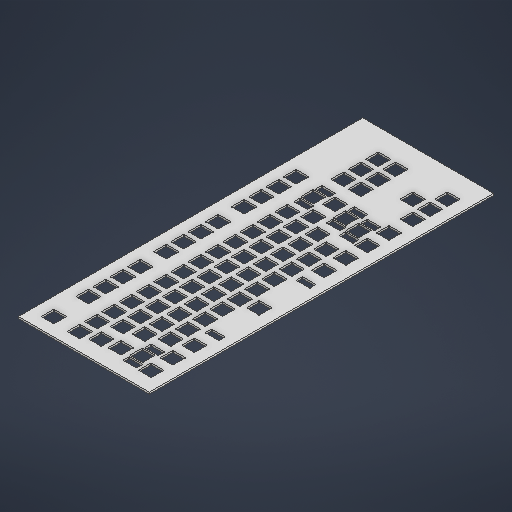
# Autodesk Inventor part: Keyboard-top
Saved by Autodesk Inventor 2026.1 (Build 301233000, 233)
## iProperties
Created: 2025-12-15
Part Number: Keyboard-top
Material: Generic
Document SubType Name: Modeling
Designer: chest
Density: 1 g/cm^3
Appearance: Default
Author: chest
Autodesk Inventor part; units mm, degrees
(part 1 of 3)
ref_plane "YZ Plane" through (0, 0, 0) normal (1, 0, 0) x (0, 1, 0)
ref_plane "XZ Plane" through (0, 0, 0) normal (0, 1, 0) x (-1, 0, 0)
ref_plane "XY Plane" through (0, 0, 0) normal (0, 0, 1) x (1, 0, 0)
sketch "Block1" plane through (0, 0, 0) normal (0, 0, 1) x (1, 0, 0)
  line L0 (-130.9078, 18.9263) -> (-130.9078, 31.9263)
  line L1 (-116.9078, 18.9263) -> (-116.9078, 31.9263)
  line L2 (-130.4078, 18.4263) -> (-117.4078, 18.4263)
  line L3 (-130.4078, 32.4263) -> (-117.4078, 32.4263)
  arc A0 (-130.9078, 18.9263) -> (-130.4078, 18.4263) centre (-130.4078, 18.9263) ccw
  arc A1 (-130.4078, 32.4263) -> (-130.9078, 31.9263) centre (-130.4078, 31.9263) ccw
  arc A2 (-117.4078, 18.4263) -> (-116.9078, 18.9263) centre (-117.4078, 18.9263) ccw
  arc A3 (-116.9078, 31.9263) -> (-117.4078, 32.4263) centre (-117.4078, 31.9263) ccw
  line L4 (-130.9078, 57.0263) -> (-130.9078, 70.0263)
  line L5 (-116.9078, 57.0263) -> (-116.9078, 70.0263)
  line L6 (-130.4078, 56.5263) -> (-117.4078, 56.5263)
  line L7 (-130.4078, 70.5263) -> (-117.4078, 70.5263)
  arc A4 (-130.9078, 57.0263) -> (-130.4078, 56.5263) centre (-130.4078, 57.0263) ccw
  arc A5 (-130.4078, 70.5263) -> (-130.9078, 70.0263) centre (-130.4078, 70.0263) ccw
  arc A6 (-117.4078, 56.5263) -> (-116.9078, 57.0263) centre (-117.4078, 57.0263) ccw
  arc A7 (-116.9078, 70.0263) -> (-117.4078, 70.5263) centre (-117.4078, 70.0263) ccw
  line L8 (-130.9078, 76.0763) -> (-130.9078, 89.0763)
  line L9 (-116.9078, 76.0763) -> (-116.9078, 89.0763)
  line L10 (-130.4078, 75.5763) -> (-117.4078, 75.5763)
  line L11 (-130.4078, 89.5763) -> (-117.4078, 89.5763)
  arc A8 (-130.9078, 76.0763) -> (-130.4078, 75.5763) centre (-130.4078, 76.0763) ccw
  arc A9 (-130.4078, 89.5763) -> (-130.9078, 89.0763) centre (-130.4078, 89.0763) ccw
  arc A10 (-117.4078, 75.5763) -> (-116.9078, 76.0763) centre (-117.4078, 76.0763) ccw
  arc A11 (-116.9078, 89.0763) -> (-117.4078, 89.5763) centre (-117.4078, 89.0763) ccw
  line L12 (-130.9078, 95.1263) -> (-130.9078, 108.1263)
  line L13 (-116.9078, 95.1263) -> (-116.9078, 108.1263)
  line L14 (-130.4078, 94.6263) -> (-117.4078, 94.6263)
  line L15 (-130.4078, 108.6263) -> (-117.4078, 108.6263)
  arc A12 (-130.9078, 95.1263) -> (-130.4078, 94.6263) centre (-130.4078, 95.1263) ccw
  arc A13 (-130.4078, 108.6263) -> (-130.9078, 108.1263) centre (-130.4078, 108.1263) ccw
  arc A14 (-117.4078, 94.6263) -> (-116.9078, 95.1263) centre (-117.4078, 95.1263) ccw
  arc A15 (-116.9078, 108.1263) -> (-117.4078, 108.6263) centre (-117.4078, 108.1263) ccw
  line L16 (-130.9078, 114.1763) -> (-130.9078, 127.1763)
  line L17 (-116.9078, 114.1763) -> (-116.9078, 127.1763)
  line L18 (-130.4078, 113.6763) -> (-117.4078, 113.6763)
  line L19 (-130.4078, 127.6763) -> (-117.4078, 127.6763)
  arc A16 (-130.9078, 114.1763) -> (-130.4078, 113.6763) centre (-130.4078, 114.1763) ccw
  arc A17 (-130.4078, 127.6763) -> (-130.9078, 127.1763) centre (-130.4078, 127.1763) ccw
  arc A18 (-117.4078, 113.6763) -> (-116.9078, 114.1763) centre (-117.4078, 114.1763) ccw
  arc A19 (-116.9078, 127.1763) -> (-117.4078, 127.6763) centre (-117.4078, 127.1763) ccw
  line L20 (-130.9078, 142.7513) -> (-130.9078, 155.7513)
  line L21 (-116.9078, 142.7513) -> (-116.9078, 155.7513)
  line L22 (-130.4078, 142.2513) -> (-117.4078, 142.2513)
  line L23 (-130.4078, 156.2513) -> (-117.4078, 156.2513)
  arc A20 (-130.9078, 142.7513) -> (-130.4078, 142.2513) centre (-130.4078, 142.7513) ccw
  arc A21 (-130.4078, 156.2513) -> (-130.9078, 155.7513) centre (-130.4078, 155.7513) ccw
  arc A22 (-117.4078, 142.2513) -> (-116.9078, 142.7513) centre (-117.4078, 142.7513) ccw
  arc A23 (-116.9078, 155.7513) -> (-117.4078, 156.2513) centre (-117.4078, 155.7513) ccw
  line L24 (-130.9078, 161.8013) -> (-130.9078, 174.8013)
  line L25 (-116.9078, 161.8013) -> (-116.9078, 174.8013)
  line L26 (-130.4078, 161.3013) -> (-117.4078, 161.3013)
  line L27 (-130.4078, 175.3013) -> (-117.4078, 175.3013)
  arc A24 (-130.9078, 161.8013) -> (-130.4078, 161.3013) centre (-130.4078, 161.8013) ccw
  arc A25 (-130.4078, 175.3013) -> (-130.9078, 174.8013) centre (-130.4078, 174.8013) ccw
  arc A26 (-117.4078, 161.3013) -> (-116.9078, 161.8013) centre (-117.4078, 161.8013) ccw
  arc A27 (-116.9078, 174.8013) -> (-117.4078, 175.3013) centre (-117.4078, 174.8013) ccw
  line L28 (-130.9078, 180.8513) -> (-130.9078, 193.8513)
  line L29 (-116.9078, 180.8513) -> (-116.9078, 193.8513)
  line L30 (-130.4078, 180.3513) -> (-117.4078, 180.3513)
  line L31 (-130.4078, 194.3513) -> (-117.4078, 194.3513)
  arc A28 (-130.9078, 180.8513) -> (-130.4078, 180.3513) centre (-130.4078, 180.8513) ccw
  arc A29 (-130.4078, 194.3513) -> (-130.9078, 193.8513) centre (-130.4078, 193.8513) ccw
  arc A30 (-117.4078, 180.3513) -> (-116.9078, 180.8513) centre (-117.4078, 180.8513) ccw
  arc A31 (-116.9078, 193.8513) -> (-117.4078, 194.3513) centre (-117.4078, 193.8513) ccw
  line L32 (-130.9078, 199.9013) -> (-130.9078, 212.9013)
  line L33 (-116.9078, 199.9013) -> (-116.9078, 212.9013)
  line L34 (-130.4078, 199.4013) -> (-117.4078, 199.4013)
  line L35 (-130.4078, 213.4013) -> (-117.4078, 213.4013)
  arc A32 (-130.9078, 199.9013) -> (-130.4078, 199.4013) centre (-130.4078, 199.9013) ccw
  arc A33 (-130.4078, 213.4013) -> (-130.9078, 212.9013) centre (-130.4078, 212.9013) ccw
  arc A34 (-117.4078, 199.4013) -> (-116.9078, 199.9013) centre (-117.4078, 199.9013) ccw
  arc A35 (-116.9078, 212.9013) -> (-117.4078, 213.4013) centre (-117.4078, 212.9013) ccw
  line L36 (-130.9078, 228.4763) -> (-130.9078, 241.4763)
  line L37 (-116.9078, 228.4763) -> (-116.9078, 241.4763)
  line L38 (-130.4078, 227.9763) -> (-117.4078, 227.9763)
  line L39 (-130.4078, 241.9763) -> (-117.4078, 241.9763)
  arc A36 (-130.9078, 228.4763) -> (-130.4078, 227.9763) centre (-130.4078, 228.4763) ccw
  arc A37 (-130.4078, 241.9763) -> (-130.9078, 241.4763) centre (-130.4078, 241.4763) ccw
  arc A38 (-117.4078, 227.9763) -> (-116.9078, 228.4763) centre (-117.4078, 228.4763) ccw
  arc A39 (-116.9078, 241.4763) -> (-117.4078, 241.9763) centre (-117.4078, 241.4763) ccw
  line L40 (-130.9078, 247.5263) -> (-130.9078, 260.5263)
  line L41 (-116.9078, 247.5263) -> (-116.9078, 260.5263)
  line L42 (-130.4078, 247.0263) -> (-117.4078, 247.0263)
  line L43 (-130.4078, 261.0263) -> (-117.4078, 261.0263)
  arc A40 (-130.9078, 247.5263) -> (-130.4078, 247.0263) centre (-130.4078, 247.5263) ccw
  arc A41 (-130.4078, 261.0263) -> (-130.9078, 260.5263) centre (-130.4078, 260.5263) ccw
  arc A42 (-117.4078, 247.0263) -> (-116.9078, 247.5263) centre (-117.4078, 247.5263) ccw
  arc A43 (-116.9078, 260.5263) -> (-117.4078, 261.0263) centre (-117.4078, 260.5263) ccw
  line L44 (-130.9078, 266.5763) -> (-130.9078, 279.5763)
  line L45 (-116.9078, 266.5763) -> (-116.9078, 279.5763)
  line L46 (-130.4078, 266.0763) -> (-117.4078, 266.0763)
  line L47 (-130.4078, 280.0763) -> (-117.4078, 280.0763)
  arc A44 (-130.9078, 266.5763) -> (-130.4078, 266.0763) centre (-130.4078, 266.5763) ccw
  arc A45 (-130.4078, 280.0763) -> (-130.9078, 279.5763) centre (-130.4078, 279.5763) ccw
  arc A46 (-117.4078, 266.0763) -> (-116.9078, 266.5763) centre (-117.4078, 266.5763) ccw
  arc A47 (-116.9078, 279.5763) -> (-117.4078, 280.0763) centre (-117.4078, 279.5763) ccw
  line L48 (-130.9078, 285.6263) -> (-130.9078, 298.6263)
  line L49 (-116.9078, 285.6263) -> (-116.9078, 298.6263)
  line L50 (-130.4078, 285.1263) -> (-117.4078, 285.1263)
  line L51 (-130.4078, 299.1263) -> (-117.4078, 299.1263)
  arc A48 (-130.9078, 285.6263) -> (-130.4078, 285.1263) centre (-130.4078, 285.6263) ccw
  arc A49 (-130.4078, 299.1263) -> (-130.9078, 298.6263) centre (-130.4078, 298.6263) ccw
  arc A50 (-117.4078, 285.1263) -> (-116.9078, 285.6263) centre (-117.4078, 285.6263) ccw
  arc A51 (-116.9078, 298.6263) -> (-117.4078, 299.1263) centre (-117.4078, 298.6263) ccw
  line L52 (-102.3328, 18.9263) -> (-102.3328, 31.9263)
  line L53 (-88.3328, 18.9263) -> (-88.3328, 31.9263)
  line L54 (-101.8328, 18.4263) -> (-88.8328, 18.4263)
  line L55 (-101.8328, 32.4263) -> (-88.8328, 32.4263)
  arc A52 (-102.3328, 18.9263) -> (-101.8328, 18.4263) centre (-101.8328, 18.9263) ccw
  arc A53 (-101.8328, 32.4263) -> (-102.3328, 31.9263) centre (-101.8328, 31.9263) ccw
  arc A54 (-88.8328, 18.4263) -> (-88.3328, 18.9263) centre (-88.8328, 18.9263) ccw
  arc A55 (-88.3328, 31.9263) -> (-88.8328, 32.4263) centre (-88.8328, 31.9263) ccw
  line L56 (-102.3328, 37.9763) -> (-102.3328, 50.9763)
  line L57 (-88.3328, 37.9763) -> (-88.3328, 50.9763)
  line L58 (-101.8328, 37.4763) -> (-88.8328, 37.4763)
  line L59 (-101.8328, 51.4763) -> (-88.8328, 51.4763)
  arc A56 (-102.3328, 37.9763) -> (-101.8328, 37.4763) centre (-101.8328, 37.9763) ccw
  arc A57 (-101.8328, 51.4763) -> (-102.3328, 50.9763) centre (-101.8328, 50.9763) ccw
  arc A58 (-88.8328, 37.4763) -> (-88.3328, 37.9763) centre (-88.8328, 37.9763) ccw
  arc A59 (-88.3328, 50.9763) -> (-88.8328, 51.4763) centre (-88.8328, 50.9763) ccw
  line L60 (-102.3328, 57.0263) -> (-102.3328, 70.0263)
  line L61 (-88.3328, 57.0263) -> (-88.3328, 70.0263)
  line L62 (-101.8328, 56.5263) -> (-88.8328, 56.5263)
  line L63 (-101.8328, 70.5263) -> (-88.8328, 70.5263)
  arc A60 (-102.3328, 57.0263) -> (-101.8328, 56.5263) centre (-101.8328, 57.0263) ccw
  arc A61 (-101.8328, 70.5263) -> (-102.3328, 70.0263) centre (-101.8328, 70.0263) ccw
  arc A62 (-88.8328, 56.5263) -> (-88.3328, 57.0263) centre (-88.8328, 57.0263) ccw
  arc A63 (-88.3328, 70.0263) -> (-88.8328, 70.5263) centre (-88.8328, 70.0263) ccw
  line L64 (-102.3328, 76.0763) -> (-102.3328, 89.0763)
  line L65 (-88.3328, 76.0763) -> (-88.3328, 89.0763)
  line L66 (-101.8328, 75.5763) -> (-88.8328, 75.5763)
  line L67 (-101.8328, 89.5763) -> (-88.8328, 89.5763)
  arc A64 (-102.3328, 76.0763) -> (-101.8328, 75.5763) centre (-101.8328, 76.0763) ccw
  arc A65 (-101.8328, 89.5763) -> (-102.3328, 89.0763) centre (-101.8328, 89.0763) ccw
  arc A66 (-88.8328, 75.5763) -> (-88.3328, 76.0763) centre (-88.8328, 76.0763) ccw
  arc A67 (-88.3328, 89.0763) -> (-88.8328, 89.5763) centre (-88.8328, 89.0763) ccw
  line L68 (-102.3328, 95.1263) -> (-102.3328, 108.1263)
  line L69 (-88.3328, 95.1263) -> (-88.3328, 108.1263)
  line L70 (-101.8328, 94.6263) -> (-88.8328, 94.6263)
  line L71 (-101.8328, 108.6263) -> (-88.8328, 108.6263)
  arc A68 (-102.3328, 95.1263) -> (-101.8328, 94.6263) centre (-101.8328, 95.1263) ccw
  arc A69 (-101.8328, 108.6263) -> (-102.3328, 108.1263) centre (-101.8328, 108.1263) ccw
  arc A70 (-88.8328, 94.6263) -> (-88.3328, 95.1263) centre (-88.8328, 95.1263) ccw
  arc A71 (-88.3328, 108.1263) -> (-88.8328, 108.6263) centre (-88.8328, 108.1263) ccw
  line L72 (-102.3328, 114.1763) -> (-102.3328, 127.1763)
  line L73 (-88.3328, 114.1763) -> (-88.3328, 127.1763)
  line L74 (-101.8328, 113.6763) -> (-88.8328, 113.6763)
  line L75 (-101.8328, 127.6763) -> (-88.8328, 127.6763)
  arc A72 (-102.3328, 114.1763) -> (-101.8328, 113.6763) centre (-101.8328, 114.1763) ccw
  arc A73 (-101.8328, 127.6763) -> (-102.3328, 127.1763) centre (-101.8328, 127.1763) ccw
  arc A74 (-88.8328, 113.6763) -> (-88.3328, 114.1763) centre (-88.8328, 114.1763) ccw
  arc A75 (-88.3328, 127.1763) -> (-88.8328, 127.6763) centre (-88.8328, 127.1763) ccw
  line L76 (-102.3328, 133.2263) -> (-102.3328, 146.2263)
  line L77 (-88.3328, 133.2263) -> (-88.3328, 146.2263)
  line L78 (-101.8328, 132.7263) -> (-88.8328, 132.7263)
  line L79 (-101.8328, 146.7263) -> (-88.8328, 146.7263)
  arc A76 (-102.3328, 133.2263) -> (-101.8328, 132.7263) centre (-101.8328, 133.2263) ccw
  arc A77 (-101.8328, 146.7263) -> (-102.3328, 146.2263) centre (-101.8328, 146.2263) ccw
  arc A78 (-88.8328, 132.7263) -> (-88.3328, 133.2263) centre (-88.8328, 133.2263) ccw
  arc A79 (-88.3328, 146.2263) -> (-88.8328, 146.7263) centre (-88.8328, 146.2263) ccw
  line L80 (-102.3328, 152.2763) -> (-102.3328, 165.2763)
  line L81 (-88.3328, 152.2763) -> (-88.3328, 165.2763)
  line L82 (-101.8328, 151.7763) -> (-88.8328, 151.7763)
  line L83 (-101.8328, 165.7763) -> (-88.8328, 165.7763)
  arc A80 (-102.3328, 152.2763) -> (-101.8328, 151.7763) centre (-101.8328, 152.2763) ccw
  arc A81 (-101.8328, 165.7763) -> (-102.3328, 165.2763) centre (-101.8328, 165.2763) ccw
  arc A82 (-88.8328, 151.7763) -> (-88.3328, 152.2763) centre (-88.8328, 152.2763) ccw
  arc A83 (-88.3328, 165.2763) -> (-88.8328, 165.7763) centre (-88.8328, 165.2763) ccw
  line L84 (-102.3328, 171.3263) -> (-102.3328, 184.3263)
  line L85 (-88.3328, 171.3263) -> (-88.3328, 184.3263)
  line L86 (-101.8328, 170.8263) -> (-88.8328, 170.8263)
  line L87 (-101.8328, 184.8263) -> (-88.8328, 184.8263)
  arc A84 (-102.3328, 171.3263) -> (-101.8328, 170.8263) centre (-101.8328, 171.3263) ccw
  arc A85 (-101.8328, 184.8263) -> (-102.3328, 184.3263) centre (-101.8328, 184.3263) ccw
  arc A86 (-88.8328, 170.8263) -> (-88.3328, 171.3263) centre (-88.8328, 171.3263) ccw
  arc A87 (-88.3328, 184.3263) -> (-88.8328, 184.8263) centre (-88.8328, 184.3263) ccw
  line L88 (-102.3328, 190.3763) -> (-102.3328, 203.3763)
  line L89 (-88.3328, 190.3763) -> (-88.3328, 203.3763)
  line L90 (-101.8328, 189.8763) -> (-88.8328, 189.8763)
  line L91 (-101.8328, 203.8763) -> (-88.8328, 203.8763)
  arc A88 (-102.3328, 190.3763) -> (-101.8328, 189.8763) centre (-101.8328, 190.3763) ccw
  arc A89 (-101.8328, 203.8763) -> (-102.3328, 203.3763) centre (-101.8328, 203.3763) ccw
  arc A90 (-88.8328, 189.8763) -> (-88.3328, 190.3763) centre (-88.8328, 190.3763) ccw
  arc A91 (-88.3328, 203.3763) -> (-88.8328, 203.8763) centre (-88.8328, 203.3763) ccw
  line L92 (-102.3328, 209.4263) -> (-102.3328, 222.4263)
  line L93 (-88.3328, 209.4263) -> (-88.3328, 222.4263)
  line L94 (-101.8328, 208.9263) -> (-88.8328, 208.9263)
  line L95 (-101.8328, 222.9263) -> (-88.8328, 222.9263)
  arc A92 (-102.3328, 209.4263) -> (-101.8328, 208.9263) centre (-101.8328, 209.4263) ccw
  arc A93 (-101.8328, 222.9263) -> (-102.3328, 222.4263) centre (-101.8328, 222.4263) ccw
  arc A94 (-88.8328, 208.9263) -> (-88.3328, 209.4263) centre (-88.8328, 209.4263) ccw
  arc A95 (-88.3328, 222.4263) -> (-88.8328, 222.9263) centre (-88.8328, 222.4263) ccw
  line L96 (-102.3328, 228.4763) -> (-102.3328, 241.4763)
  line L97 (-88.3328, 228.4763) -> (-88.3328, 241.4763)
  line L98 (-101.8328, 227.9763) -> (-88.8328, 227.9763)
  line L99 (-101.8328, 241.9763) -> (-88.8328, 241.9763)
  arc A96 (-102.3328, 228.4763) -> (-101.8328, 227.9763) centre (-101.8328, 228.4763) ccw
  arc A97 (-101.8328, 241.9763) -> (-102.3328, 241.4763) centre (-101.8328, 241.4763) ccw
  arc A98 (-88.8328, 227.9763) -> (-88.3328, 228.4763) centre (-88.8328, 228.4763) ccw
  arc A99 (-88.3328, 241.4763) -> (-88.8328, 241.9763) centre (-88.8328, 241.4763) ccw
  line L100 (-102.3328, 247.5263) -> (-102.3328, 260.5263)
  line L101 (-88.3328, 247.5263) -> (-88.3328, 260.5263)
  line L102 (-101.8328, 247.0263) -> (-88.8328, 247.0263)
  line L103 (-101.8328, 261.0263) -> (-88.8328, 261.0263)
  arc A100 (-102.3328, 247.5263) -> (-101.8328, 247.0263) centre (-101.8328, 247.5263) ccw
  arc A101 (-101.8328, 261.0263) -> (-102.3328, 260.5263) centre (-101.8328, 260.5263) ccw
  arc A102 (-88.8328, 247.0263) -> (-88.3328, 247.5263) centre (-88.8328, 247.5263) ccw
  arc A103 (-88.3328, 260.5263) -> (-88.8328, 261.0263) centre (-88.8328, 260.5263) ccw
  line L104 (-102.3328, 276.1013) -> (-102.3328, 289.1013)
  line L105 (-88.3328, 276.1013) -> (-88.3328, 289.1013)
  line L106 (-101.8328, 275.6013) -> (-88.8328, 275.6013)
  line L107 (-101.8328, 289.6013) -> (-88.8328, 289.6013)
  arc A104 (-102.3328, 276.1013) -> (-101.8328, 275.6013) centre (-101.8328, 276.1013) ccw
  arc A105 (-101.8328, 289.6013) -> (-102.3328, 289.1013) centre (-101.8328, 289.1013) ccw
  arc A106 (-88.8328, 275.6013) -> (-88.3328, 276.1013) centre (-88.8328, 276.1013) ccw
  arc A107 (-88.3328, 289.1013) -> (-88.8328, 289.6013) centre (-88.8328, 289.1013) ccw
  line L108 (-101.3328, 267.6633) -> (-101.3328, 273.6633)
  line L109 (-86.3328, 267.6633) -> (-86.3328, 273.6633)
  line L110 (-100.8328, 267.1633) -> (-86.8328, 267.1633)
  line L111 (-100.8328, 274.1633) -> (-86.8328, 274.1633)
  arc A108 (-101.3328, 267.6633) -> (-100.8328, 267.1633) centre (-100.8328, 267.6633) ccw
  arc A109 (-100.8328, 274.1633) -> (-101.3328, 273.6633) centre (-100.8328, 273.6633) ccw
  arc A110 (-86.8328, 267.1633) -> (-86.3328, 267.6633) centre (-86.8328, 267.6633) ccw
  arc A111 (-86.3328, 273.6633) -> (-86.8328, 274.1633) centre (-86.8328, 273.6633) ccw
  line L112 (-101.3328, 291.5393) -> (-101.3328, 297.5393)
  line L113 (-86.3328, 291.5393) -> (-86.3328, 297.5393)
  line L114 (-100.8328, 291.0393) -> (-86.8328, 291.0393)
  line L115 (-100.8328, 298.0393) -> (-86.8328, 298.0393)
  arc A112 (-101.3328, 291.5393) -> (-100.8328, 291.0393) centre (-100.8328, 291.5393) ccw
  arc A113 (-100.8328, 298.0393) -> (-101.3328, 297.5393) centre (-100.8328, 297.5393) ccw
  arc A114 (-86.8328, 291.0393) -> (-86.3328, 291.5393) centre (-86.8328, 291.5393) ccw
  arc A115 (-86.3328, 297.5393) -> (-86.8328, 298.0393) centre (-86.8328, 297.5393) ccw
  line L116 (-102.3328, 309.4388) -> (-102.3328, 322.4388)
  line L117 (-88.3328, 309.4388) -> (-88.3328, 322.4388)
  line L118 (-101.8328, 308.9388) -> (-88.8328, 308.9388)
  line L119 (-101.8328, 322.9388) -> (-88.8328, 322.9388)
  arc A116 (-102.3328, 309.4388) -> (-101.8328, 308.9388) centre (-101.8328, 309.4388) ccw
  arc A117 (-101.8328, 322.9388) -> (-102.3328, 322.4388) centre (-101.8328, 322.4388) ccw
  arc A118 (-88.8328, 308.9388) -> (-88.3328, 309.4388) centre (-88.8328, 309.4388) ccw
  arc A119 (-88.3328, 322.4388) -> (-88.8328, 322.9388) centre (-88.8328, 322.4388) ccw
  line L120 (-102.3328, 328.4888) -> (-102.3328, 341.4888)
  line L121 (-88.3328, 328.4888) -> (-88.3328, 341.4888)
  line L122 (-101.8328, 327.9888) -> (-88.8328, 327.9888)
  line L123 (-101.8328, 341.9888) -> (-88.8328, 341.9888)
  arc A120 (-102.3328, 328.4888) -> (-101.8328, 327.9888) centre (-101.8328, 328.4888) ccw
  arc A121 (-101.8328, 341.9888) -> (-102.3328, 341.4888) centre (-101.8328, 341.4888) ccw
  arc A122 (-88.8328, 327.9888) -> (-88.3328, 328.4888) centre (-88.8328, 328.4888) ccw
  arc A123 (-88.3328, 341.4888) -> (-88.8328, 341.9888) centre (-88.8328, 341.4888) ccw
  line L124 (-102.3328, 347.5388) -> (-102.3328, 360.5388)
  line L125 (-88.3328, 347.5388) -> (-88.3328, 360.5388)
  line L126 (-101.8328, 347.0388) -> (-88.8328, 347.0388)
  line L127 (-101.8328, 361.0388) -> (-88.8328, 361.0388)
  arc A124 (-102.3328, 347.5388) -> (-101.8328, 347.0388) centre (-101.8328, 347.5388) ccw
  arc A125 (-101.8328, 361.0388) -> (-102.3328, 360.5388) centre (-101.8328, 360.5388) ccw
  arc A126 (-88.8328, 347.0388) -> (-88.3328, 347.5388) centre (-88.8328, 347.5388) ccw
  arc A127 (-88.3328, 360.5388) -> (-88.8328, 361.0388) centre (-88.8328, 360.5388) ccw
  line L128 (-83.2828, 23.6888) -> (-83.2828, 36.6888)
  line L129 (-69.2828, 23.6888) -> (-69.2828, 36.6888)
  line L130 (-82.7828, 23.1888) -> (-69.7828, 23.1888)
  line L131 (-82.7828, 37.1888) -> (-69.7828, 37.1888)
  arc A128 (-83.2828, 23.6888) -> (-82.7828, 23.1888) centre (-82.7828, 23.6888) ccw
  arc A129 (-82.7828, 37.1888) -> (-83.2828, 36.6888) centre (-82.7828, 36.6888) ccw
  arc A130 (-69.7828, 23.1888) -> (-69.2828, 23.6888) centre (-69.7828, 23.6888) ccw
  arc A131 (-69.2828, 36.6888) -> (-69.7828, 37.1888) centre (-69.7828, 36.6888) ccw
  line L132 (-83.2828, 47.5013) -> (-83.2828, 60.5013)
  line L133 (-69.2828, 47.5013) -> (-69.2828, 60.5013)
  line L134 (-82.7828, 47.0013) -> (-69.7828, 47.0013)
  line L135 (-82.7828, 61.0013) -> (-69.7828, 61.0013)
  arc A132 (-83.2828, 47.5013) -> (-82.7828, 47.0013) centre (-82.7828, 47.5013) ccw
  arc A133 (-82.7828, 61.0013) -> (-83.2828, 60.5013) centre (-82.7828, 60.5013) ccw
  arc A134 (-69.7828, 47.0013) -> (-69.2828, 47.5013) centre (-69.7828, 47.5013) ccw
  arc A135 (-69.2828, 60.5013) -> (-69.7828, 61.0013) centre (-69.7828, 60.5013) ccw
  line L136 (-83.2828, 66.5513) -> (-83.2828, 79.5513)
  line L137 (-69.2828, 66.5513) -> (-69.2828, 79.5513)
  line L138 (-82.7828, 66.0513) -> (-69.7828, 66.0513)
  line L139 (-82.7828, 80.0513) -> (-69.7828, 80.0513)
  arc A136 (-83.2828, 66.5513) -> (-82.7828, 66.0513) centre (-82.7828, 66.5513) ccw
  arc A137 (-82.7828, 80.0513) -> (-83.2828, 79.5513) centre (-82.7828, 79.5513) ccw
  arc A138 (-69.7828, 66.0513) -> (-69.2828, 66.5513) centre (-69.7828, 66.5513) ccw
  arc A139 (-69.2828, 79.5513) -> (-69.7828, 80.0513) centre (-69.7828, 79.5513) ccw
  line L140 (-83.2828, 85.6013) -> (-83.2828, 98.6013)
  line L141 (-69.2828, 85.6013) -> (-69.2828, 98.6013)
  line L142 (-82.7828, 85.1013) -> (-69.7828, 85.1013)
  line L143 (-82.7828, 99.1013) -> (-69.7828, 99.1013)
  arc A140 (-83.2828, 85.6013) -> (-82.7828, 85.1013) centre (-82.7828, 85.6013) ccw
  arc A141 (-82.7828, 99.1013) -> (-83.2828, 98.6013) centre (-82.7828, 98.6013) ccw
  arc A142 (-69.7828, 85.1013) -> (-69.2828, 85.6013) centre (-69.7828, 85.6013) ccw
  arc A143 (-69.2828, 98.6013) -> (-69.7828, 99.1013) centre (-69.7828, 98.6013) ccw
  line L144 (-83.2828, 104.6513) -> (-83.2828, 117.6513)
  line L145 (-69.2828, 104.6513) -> (-69.2828, 117.6513)
  line L146 (-82.7828, 104.1513) -> (-69.7828, 104.1513)
  line L147 (-82.7828, 118.1513) -> (-69.7828, 118.1513)
  arc A144 (-83.2828, 104.6513) -> (-82.7828, 104.1513) centre (-82.7828, 104.6513) ccw
  arc A145 (-82.7828, 118.1513) -> (-83.2828, 117.6513) centre (-82.7828, 117.6513) ccw
  arc A146 (-69.7828, 104.1513) -> (-69.2828, 104.6513) centre (-69.7828, 104.6513) ccw
  arc A147 (-69.2828, 117.6513) -> (-69.7828, 118.1513) centre (-69.7828, 117.6513) ccw
  line L148 (-83.2828, 123.7013) -> (-83.2828, 136.7013)
  line L149 (-69.2828, 123.7013) -> (-69.2828, 136.7013)
  line L150 (-82.7828, 123.2013) -> (-69.7828, 123.2013)
  line L151 (-82.7828, 137.2013) -> (-69.7828, 137.2013)
  arc A148 (-83.2828, 123.7013) -> (-82.7828, 123.2013) centre (-82.7828, 123.7013) ccw
  arc A149 (-82.7828, 137.2013) -> (-83.2828, 136.7013) centre (-82.7828, 136.7013) ccw
  arc A150 (-69.7828, 123.2013) -> (-69.2828, 123.7013) centre (-69.7828, 123.7013) ccw
  arc A151 (-69.2828, 136.7013) -> (-69.7828, 137.2013) centre (-69.7828, 136.7013) ccw
  line L152 (-83.2828, 142.7513) -> (-83.2828, 155.7513)
  line L153 (-69.2828, 142.7513) -> (-69.2828, 155.7513)
  line L154 (-82.7828, 142.2513) -> (-69.7828, 142.2513)
  line L155 (-82.7828, 156.2513) -> (-69.7828, 156.2513)
  arc A152 (-83.2828, 142.7513) -> (-82.7828, 142.2513) centre (-82.7828, 142.7513) ccw
  arc A153 (-82.7828, 156.2513) -> (-83.2828, 155.7513) centre (-82.7828, 155.7513) ccw
  arc A154 (-69.7828, 142.2513) -> (-69.2828, 142.7513) centre (-69.7828, 142.7513) ccw
  arc A155 (-69.2828, 155.7513) -> (-69.7828, 156.2513) centre (-69.7828, 155.7513) ccw
  line L156 (-83.2828, 161.8013) -> (-83.2828, 174.8013)
  line L157 (-69.2828, 161.8013) -> (-69.2828, 174.8013)
  line L158 (-82.7828, 161.3013) -> (-69.7828, 161.3013)
  line L159 (-82.7828, 175.3013) -> (-69.7828, 175.3013)
  arc A156 (-83.2828, 161.8013) -> (-82.7828, 161.3013) centre (-82.7828, 161.8013) ccw
  arc A157 (-82.7828, 175.3013) -> (-83.2828, 174.8013) centre (-82.7828, 174.8013) ccw
  arc A158 (-69.7828, 161.3013) -> (-69.2828, 161.8013) centre (-69.7828, 161.8013) ccw
  arc A159 (-69.2828, 174.8013) -> (-69.7828, 175.3013) centre (-69.7828, 174.8013) ccw
  line L160 (-83.2828, 180.8513) -> (-83.2828, 193.8513)
  line L161 (-69.2828, 180.8513) -> (-69.2828, 193.8513)
  line L162 (-82.7828, 180.3513) -> (-69.7828, 180.3513)
  line L163 (-82.7828, 194.3513) -> (-69.7828, 194.3513)
  arc A160 (-83.2828, 180.8513) -> (-82.7828, 180.3513) centre (-82.7828, 180.8513) ccw
  arc A161 (-82.7828, 194.3513) -> (-83.2828, 193.8513) centre (-82.7828, 193.8513) ccw
  arc A162 (-69.7828, 180.3513) -> (-69.2828, 180.8513) centre (-69.7828, 180.8513) ccw
  arc A163 (-69.2828, 193.8513) -> (-69.7828, 194.3513) centre (-69.7828, 193.8513) ccw
  line L164 (-83.2828, 199.9013) -> (-83.2828, 212.9013)
  line L165 (-69.2828, 199.9013) -> (-69.2828, 212.9013)
  line L166 (-82.7828, 199.4013) -> (-69.7828, 199.4013)
  line L167 (-82.7828, 213.4013) -> (-69.7828, 213.4013)
  arc A164 (-83.2828, 199.9013) -> (-82.7828, 199.4013) centre (-82.7828, 199.9013) ccw
  arc A165 (-82.7828, 213.4013) -> (-83.2828, 212.9013) centre (-82.7828, 212.9013) ccw
  arc A166 (-69.7828, 199.4013) -> (-69.2828, 199.9013) centre (-69.7828, 199.9013) ccw
  arc A167 (-69.2828, 212.9013) -> (-69.7828, 213.4013) centre (-69.7828, 212.9013) ccw
  line L168 (-83.2828, 218.9513) -> (-83.2828, 231.9513)
  line L169 (-69.2828, 218.9513) -> (-69.2828, 231.9513)
  line L170 (-82.7828, 218.4513) -> (-69.7828, 218.4513)
  line L171 (-82.7828, 232.4513) -> (-69.7828, 232.4513)
  arc A168 (-83.2828, 218.9513) -> (-82.7828, 218.4513) centre (-82.7828, 218.9513) ccw
  arc A169 (-82.7828, 232.4513) -> (-83.2828, 231.9513) centre (-82.7828, 231.9513) ccw
  arc A170 (-69.7828, 218.4513) -> (-69.2828, 218.9513) centre (-69.7828, 218.9513) ccw
  arc A171 (-69.2828, 231.9513) -> (-69.7828, 232.4513) centre (-69.7828, 231.9513) ccw
  line L172 (-83.2828, 238.0013) -> (-83.2828, 251.0013)
  line L173 (-69.2828, 238.0013) -> (-69.2828, 251.0013)
  line L174 (-82.7828, 237.5013) -> (-69.7828, 237.5013)
  line L175 (-82.7828, 251.5013) -> (-69.7828, 251.5013)
  arc A172 (-83.2828, 238.0013) -> (-82.7828, 237.5013) centre (-82.7828, 238.0013) ccw
  arc A173 (-82.7828, 251.5013) -> (-83.2828, 251.0013) centre (-82.7828, 251.0013) ccw
  arc A174 (-69.7828, 237.5013) -> (-69.2828, 238.0013) centre (-69.7828, 238.0013) ccw
  arc A175 (-69.2828, 251.0013) -> (-69.7828, 251.5013) centre (-69.7828, 251.0013) ccw
  line L176 (-83.2828, 257.0513) -> (-83.2828, 270.0513)
  line L177 (-69.2828, 257.0513) -> (-69.2828, 270.0513)
  line L178 (-82.7828, 256.5513) -> (-69.7828, 256.5513)
  line L179 (-82.7828, 270.5513) -> (-69.7828, 270.5513)
  arc A176 (-83.2828, 257.0513) -> (-82.7828, 256.5513) centre (-82.7828, 257.0513) ccw
  arc A177 (-82.7828, 270.5513) -> (-83.2828, 270.0513) centre (-82.7828, 270.0513) ccw
  arc A178 (-69.7828, 256.5513) -> (-69.2828, 257.0513) centre (-69.7828, 257.0513) ccw
  arc A179 (-69.2828, 270.0513) -> (-69.7828, 270.5513) centre (-69.7828, 270.0513) ccw
  line L180 (-83.2828, 280.8638) -> (-83.2828, 293.8638)
  line L181 (-69.2828, 280.8638) -> (-69.2828, 293.8638)
  line L182 (-82.7828, 280.3638) -> (-69.7828, 280.3638)
  line L183 (-82.7828, 294.3638) -> (-69.7828, 294.3638)
  arc A180 (-83.2828, 280.8638) -> (-82.7828, 280.3638) centre (-82.7828, 280.8638) ccw
  arc A181 (-82.7828, 294.3638) -> (-83.2828, 293.8638) centre (-82.7828, 293.8638) ccw
  arc A182 (-69.7828, 280.3638) -> (-69.2828, 280.8638) centre (-69.7828, 280.8638) ccw
  arc A183 (-69.2828, 293.8638) -> (-69.7828, 294.3638) centre (-69.7828, 293.8638) ccw
  line L184 (-83.2828, 309.4388) -> (-83.2828, 322.4388)
  line L185 (-69.2828, 309.4388) -> (-69.2828, 322.4388)
  line L186 (-82.7828, 308.9388) -> (-69.7828, 308.9388)
  line L187 (-82.7828, 322.9388) -> (-69.7828, 322.9388)
  arc A184 (-83.2828, 309.4388) -> (-82.7828, 308.9388) centre (-82.7828, 309.4388) ccw
  arc A185 (-82.7828, 322.9388) -> (-83.2828, 322.4388) centre (-82.7828, 322.4388) ccw
  arc A186 (-69.7828, 308.9388) -> (-69.2828, 309.4388) centre (-69.7828, 309.4388) ccw
  arc A187 (-69.2828, 322.4388) -> (-69.7828, 322.9388) centre (-69.7828, 322.4388) ccw
  line L188 (-83.2828, 328.4888) -> (-83.2828, 341.4888)
  line L189 (-69.2828, 328.4888) -> (-69.2828, 341.4888)
  line L190 (-82.7828, 327.9888) -> (-69.7828, 327.9888)
  line L191 (-82.7828, 341.9888) -> (-69.7828, 341.9888)
  arc A188 (-83.2828, 328.4888) -> (-82.7828, 327.9888) centre (-82.7828, 328.4888) ccw
  arc A189 (-82.7828, 341.9888) -> (-83.2828, 341.4888) centre (-82.7828, 341.4888) ccw
  arc A190 (-69.7828, 327.9888) -> (-69.2828, 328.4888) centre (-69.7828, 328.4888) ccw
  arc A191 (-69.2828, 341.4888) -> (-69.7828, 341.9888) centre (-69.7828, 341.4888) ccw
  line L192 (-83.2828, 347.5388) -> (-83.2828, 360.5388)
  line L193 (-69.2828, 347.5388) -> (-69.2828, 360.5388)
  line L194 (-82.7828, 347.0388) -> (-69.7828, 347.0388)
  line L195 (-82.7828, 361.0388) -> (-69.7828, 361.0388)
  arc A192 (-83.2828, 347.5388) -> (-82.7828, 347.0388) centre (-82.7828, 347.5388) ccw
  arc A193 (-82.7828, 361.0388) -> (-83.2828, 360.5388) centre (-82.7828, 360.5388) ccw
  arc A194 (-69.7828, 347.0388) -> (-69.2828, 347.5388) centre (-69.7828, 347.5388) ccw
  arc A195 (-69.2828, 360.5388) -> (-69.7828, 361.0388) centre (-69.7828, 360.5388) ccw
  line L196 (-64.2328, 26.0701) -> (-64.2328, 39.0701)
  line L197 (-50.2328, 26.0701) -> (-50.2328, 39.0701)
  line L198 (-63.7328, 25.5701) -> (-50.7328, 25.5701)
  line L199 (-63.7328, 39.5701) -> (-50.7328, 39.5701)
  arc A196 (-64.2328, 26.0701) -> (-63.7328, 25.5701) centre (-63.7328, 26.0701) ccw
  arc A197 (-63.7328, 39.5701) -> (-64.2328, 39.0701) centre (-63.7328, 39.0701) ccw
  arc A198 (-50.7328, 25.5701) -> (-50.2328, 26.0701) centre (-50.7328, 26.0701) ccw
  arc A199 (-50.2328, 39.0701) -> (-50.7328, 39.5701) centre (-50.7328, 39.0701) ccw
  line L200 (-64.2328, 52.2638) -> (-64.2328, 65.2638)
  line L201 (-50.2328, 52.2638) -> (-50.2328, 65.2638)
  line L202 (-63.7328, 51.7638) -> (-50.7328, 51.7638)
  line L203 (-63.7328, 65.7638) -> (-50.7328, 65.7638)
  arc A200 (-64.2328, 52.2638) -> (-63.7328, 51.7638) centre (-63.7328, 52.2638) ccw
  arc A201 (-63.7328, 65.7638) -> (-64.2328, 65.2638) centre (-63.7328, 65.2638) ccw
  arc A202 (-50.7328, 51.7638) -> (-50.2328, 52.2638) centre (-50.7328, 52.2638) ccw
  arc A203 (-50.2328, 65.2638) -> (-50.7328, 65.7638) centre (-50.7328, 65.2638) ccw
  line L204 (-64.2328, 71.3138) -> (-64.2328, 84.3138)
  line L205 (-50.2328, 71.3138) -> (-50.2328, 84.3138)
  line L206 (-63.7328, 70.8138) -> (-50.7328, 70.8138)
  line L207 (-63.7328, 84.8138) -> (-50.7328, 84.8138)
  arc A204 (-64.2328, 71.3138) -> (-63.7328, 70.8138) centre (-63.7328, 71.3138) ccw
  arc A205 (-63.7328, 84.8138) -> (-64.2328, 84.3138) centre (-63.7328, 84.3138) ccw
  arc A206 (-50.7328, 70.8138) -> (-50.2328, 71.3138) centre (-50.7328, 71.3138) ccw
  arc A207 (-50.2328, 84.3138) -> (-50.7328, 84.8138) centre (-50.7328, 84.3138) ccw
  line L208 (-64.2328, 90.3638) -> (-64.2328, 103.3638)
  line L209 (-50.2328, 90.3638) -> (-50.2328, 103.3638)
  line L210 (-63.7328, 89.8638) -> (-50.7328, 89.8638)
  line L211 (-63.7328, 103.8638) -> (-50.7328, 103.8638)
  arc A208 (-64.2328, 90.3638) -> (-63.7328, 89.8638) centre (-63.7328, 90.3638) ccw
  arc A209 (-63.7328, 103.8638) -> (-64.2328, 103.3638) centre (-63.7328, 103.3638) ccw
  arc A210 (-50.7328, 89.8638) -> (-50.2328, 90.3638) centre (-50.7328, 90.3638) ccw
  arc A211 (-50.2328, 103.3638) -> (-50.7328, 103.8638) centre (-50.7328, 103.3638) ccw
  line L212 (-64.2328, 109.4138) -> (-64.2328, 122.4138)
  line L213 (-50.2328, 109.4138) -> (-50.2328, 122.4138)
  line L214 (-63.7328, 108.9138) -> (-50.7328, 108.9138)
  line L215 (-63.7328, 122.9138) -> (-50.7328, 122.9138)
  arc A212 (-64.2328, 109.4138) -> (-63.7328, 108.9138) centre (-63.7328, 109.4138) ccw
  arc A213 (-63.7328, 122.9138) -> (-64.2328, 122.4138) centre (-63.7328, 122.4138) ccw
  arc A214 (-50.7328, 108.9138) -> (-50.2328, 109.4138) centre (-50.7328, 109.4138) ccw
  arc A215 (-50.2328, 122.4138) -> (-50.7328, 122.9138) centre (-50.7328, 122.4138) ccw
  line L216 (-64.2328, 128.4638) -> (-64.2328, 141.4638)
  line L217 (-50.2328, 128.4638) -> (-50.2328, 141.4638)
  line L218 (-63.7328, 127.9638) -> (-50.7328, 127.9638)
  line L219 (-63.7328, 141.9638) -> (-50.7328, 141.9638)
  arc A216 (-64.2328, 128.4638) -> (-63.7328, 127.9638) centre (-63.7328, 128.4638) ccw
  arc A217 (-63.7328, 141.9638) -> (-64.2328, 141.4638) centre (-63.7328, 141.4638) ccw
  arc A218 (-50.7328, 127.9638) -> (-50.2328, 128.4638) centre (-50.7328, 128.4638) ccw
  arc A219 (-50.2328, 141.4638) -> (-50.7328, 141.9638) centre (-50.7328, 141.4638) ccw
  line L220 (-64.2328, 147.5138) -> (-64.2328, 160.5138)
  line L221 (-50.2328, 147.5138) -> (-50.2328, 160.5138)
  line L222 (-63.7328, 147.0138) -> (-50.7328, 147.0138)
  line L223 (-63.7328, 161.0138) -> (-50.7328, 161.0138)
  arc A220 (-64.2328, 147.5138) -> (-63.7328, 147.0138) centre (-63.7328, 147.5138) ccw
  arc A221 (-63.7328, 161.0138) -> (-64.2328, 160.5138) centre (-63.7328, 160.5138) ccw
  arc A222 (-50.7328, 147.0138) -> (-50.2328, 147.5138) centre (-50.7328, 147.5138) ccw
  arc A223 (-50.2328, 160.5138) -> (-50.7328, 161.0138) centre (-50.7328, 160.5138) ccw
  line L224 (-64.2328, 166.5638) -> (-64.2328, 179.5638)
  line L225 (-50.2328, 166.5638) -> (-50.2328, 179.5638)
  line L226 (-63.7328, 166.0638) -> (-50.7328, 166.0638)
  line L227 (-63.7328, 180.0638) -> (-50.7328, 180.0638)
  arc A224 (-64.2328, 166.5638) -> (-63.7328, 166.0638) centre (-63.7328, 166.5638) ccw
  arc A225 (-63.7328, 180.0638) -> (-64.2328, 179.5638) centre (-63.7328, 179.5638) ccw
  arc A226 (-50.7328, 166.0638) -> (-50.2328, 166.5638) centre (-50.7328, 166.5638) ccw
  arc A227 (-50.2328, 179.5638) -> (-50.7328, 180.0638) centre (-50.7328, 179.5638) ccw
  line L228 (-64.2328, 185.6138) -> (-64.2328, 198.6138)
  line L229 (-50.2328, 185.6138) -> (-50.2328, 198.6138)
  line L230 (-63.7328, 185.1138) -> (-50.7328, 185.1138)
  line L231 (-63.7328, 199.1138) -> (-50.7328, 199.1138)
  arc A228 (-64.2328, 185.6138) -> (-63.7328, 185.1138) centre (-63.7328, 185.6138) ccw
  arc A229 (-63.7328, 199.1138) -> (-64.2328, 198.6138) centre (-63.7328, 198.6138) ccw
  arc A230 (-50.7328, 185.1138) -> (-50.2328, 185.6138) centre (-50.7328, 185.6138) ccw
  arc A231 (-50.2328, 198.6138) -> (-50.7328, 199.1138) centre (-50.7328, 198.6138) ccw
  line L232 (-64.2328, 204.6638) -> (-64.2328, 217.6638)
  line L233 (-50.2328, 204.6638) -> (-50.2328, 217.6638)
  line L234 (-63.7328, 204.1638) -> (-50.7328, 204.1638)
  line L235 (-63.7328, 218.1638) -> (-50.7328, 218.1638)
  arc A232 (-64.2328, 204.6638) -> (-63.7328, 204.1638) centre (-63.7328, 204.6638) ccw
  arc A233 (-63.7328, 218.1638) -> (-64.2328, 217.6638) centre (-63.7328, 217.6638) ccw
  arc A234 (-50.7328, 204.1638) -> (-50.2328, 204.6638) centre (-50.7328, 204.6638) ccw
  arc A235 (-50.2328, 217.6638) -> (-50.7328, 218.1638) centre (-50.7328, 217.6638) ccw
  line L236 (-64.2328, 223.7138) -> (-64.2328, 236.7138)
  line L237 (-50.2328, 223.7138) -> (-50.2328, 236.7138)
  line L238 (-63.7328, 223.2138) -> (-50.7328, 223.2138)
  line L239 (-63.7328, 237.2138) -> (-50.7328, 237.2138)
  arc A236 (-64.2328, 223.7138) -> (-63.7328, 223.2138) centre (-63.7328, 223.7138) ccw
  arc A237 (-63.7328, 237.2138) -> (-64.2328, 236.7138) centre (-63.7328, 236.7138) ccw
  arc A238 (-50.7328, 223.2138) -> (-50.2328, 223.7138) centre (-50.7328, 223.7138) ccw
  arc A239 (-50.2328, 236.7138) -> (-50.7328, 237.2138) centre (-50.7328, 236.7138) ccw
  line L240 (-64.2328, 242.7638) -> (-64.2328, 255.7638)
  line L241 (-50.2328, 242.7638) -> (-50.2328, 255.7638)
  line L242 (-63.7328, 242.2638) -> (-50.7328, 242.2638)
  line L243 (-63.7328, 256.2638) -> (-50.7328, 256.2638)
  arc A240 (-64.2328, 242.7638) -> (-63.7328, 242.2638) centre (-63.7328, 242.7638) ccw
  arc A241 (-63.7328, 256.2638) -> (-64.2328, 255.7638) centre (-63.7328, 255.7638) ccw
  arc A242 (-50.7328, 242.2638) -> (-50.2328, 242.7638) centre (-50.7328, 242.7638) ccw
  arc A243 (-50.2328, 255.7638) -> (-50.7328, 256.2638) centre (-50.7328, 255.7638) ccw
  line L244 (-64.2328, 273.7201) -> (-64.2328, 286.7201)
  line L245 (-50.2328, 273.7201) -> (-50.2328, 286.7201)
  line L246 (-63.7328, 273.2201) -> (-50.7328, 273.2201)
  line L247 (-63.7328, 287.2201) -> (-50.7328, 287.2201)
  arc A244 (-64.2328, 273.7201) -> (-63.7328, 273.2201) centre (-63.7328, 273.7201) ccw
  arc A245 (-63.7328, 287.2201) -> (-64.2328, 286.7201) centre (-63.7328, 286.7201) ccw
  arc A246 (-50.7328, 273.2201) -> (-50.2328, 273.7201) centre (-50.7328, 273.7201) ccw
  arc A247 (-50.2328, 286.7201) -> (-50.7328, 287.2201) centre (-50.7328, 286.7201) ccw
  line L248 (-63.2328, 265.2821) -> (-63.2328, 271.2821)
  line L249 (-48.2328, 265.2821) -> (-48.2328, 271.2821)
  line L250 (-62.7328, 264.7821) -> (-48.7328, 264.7821)
  line L251 (-62.7328, 271.7821) -> (-48.7328, 271.7821)
  arc A248 (-63.2328, 265.2821) -> (-62.7328, 264.7821) centre (-62.7328, 265.2821) ccw
  arc A249 (-62.7328, 271.7821) -> (-63.2328, 271.2821) centre (-62.7328, 271.2821) ccw
  arc A250 (-48.7328, 264.7821) -> (-48.2328, 265.2821) centre (-48.7328, 265.2821) ccw
  arc A251 (-48.2328, 271.2821) -> (-48.7328, 271.7821) centre (-48.7328, 271.2821) ccw
  line L252 (-63.2328, 289.1581) -> (-63.2328, 295.1581)
  line L253 (-48.2328, 289.1581) -> (-48.2328, 295.1581)
  line L254 (-62.7328, 288.6581) -> (-48.7328, 288.6581)
  line L255 (-62.7328, 295.6581) -> (-48.7328, 295.6581)
  arc A252 (-63.2328, 289.1581) -> (-62.7328, 288.6581) centre (-62.7328, 289.1581) ccw
  arc A253 (-62.7328, 295.6581) -> (-63.2328, 295.1581) centre (-62.7328, 295.1581) ccw
  arc A254 (-48.7328, 288.6581) -> (-48.2328, 289.1581) centre (-48.7328, 289.1581) ccw
  arc A255 (-48.2328, 295.1581) -> (-48.7328, 295.6581) centre (-48.7328, 295.1581) ccw
  line L256 (-45.1828, 30.8326) -> (-45.1828, 43.8326)
  line L257 (-31.1828, 30.8326) -> (-31.1828, 43.8326)
  line L258 (-44.6828, 30.3326) -> (-31.6828, 30.3326)
  line L259 (-44.6828, 44.3326) -> (-31.6828, 44.3326)
  arc A256 (-45.1828, 30.8326) -> (-44.6828, 30.3326) centre (-44.6828, 30.8326) ccw
  arc A257 (-44.6828, 44.3326) -> (-45.1828, 43.8326) centre (-44.6828, 43.8326) ccw
  arc A258 (-31.6828, 30.3326) -> (-31.1828, 30.8326) centre (-31.6828, 30.8326) ccw
  arc A259 (-31.1828, 43.8326) -> (-31.6828, 44.3326) centre (-31.6828, 43.8326) ccw
  line L260 (-44.1828, 22.3946) -> (-44.1828, 28.3946)
  line L261 (-29.1828, 22.3946) -> (-29.1828, 28.3946)
  line L262 (-43.6828, 21.8946) -> (-29.6828, 21.8946)
  line L263 (-43.6828, 28.8946) -> (-29.6828, 28.8946)
  arc A260 (-44.1828, 22.3946) -> (-43.6828, 21.8946) centre (-43.6828, 22.3946) ccw
  arc A261 (-43.6828, 28.8946) -> (-44.1828, 28.3946) centre (-43.6828, 28.3946) ccw
  arc A262 (-29.6828, 21.8946) -> (-29.1828, 22.3946) centre (-29.6828, 22.3946) ccw
  arc A263 (-29.1828, 28.3946) -> (-29.6828, 28.8946) centre (-29.6828, 28.3946) ccw
  line L264 (-44.1828, 46.2706) -> (-44.1828, 52.2706)
  line L265 (-29.1828, 46.2706) -> (-29.1828, 52.2706)
  line L266 (-43.6828, 45.7706) -> (-29.6828, 45.7706)
  line L267 (-43.6828, 52.7706) -> (-29.6828, 52.7706)
  arc A264 (-44.1828, 46.2706) -> (-43.6828, 45.7706) centre (-43.6828, 46.2706) ccw
  arc A265 (-43.6828, 52.7706) -> (-44.1828, 52.2706) centre (-43.6828, 52.2706) ccw
  arc A266 (-29.6828, 45.7706) -> (-29.1828, 46.2706) centre (-29.6828, 46.2706) ccw
  arc A267 (-29.1828, 52.2706) -> (-29.6828, 52.7706) centre (-29.6828, 52.2706) ccw
  line L268 (-45.1828, 61.7888) -> (-45.1828, 74.7888)
  line L269 (-31.1828, 61.7888) -> (-31.1828, 74.7888)
  line L270 (-44.6828, 61.2888) -> (-31.6828, 61.2888)
  line L271 (-44.6828, 75.2888) -> (-31.6828, 75.2888)
  arc A268 (-45.1828, 61.7888) -> (-44.6828, 61.2888) centre (-44.6828, 61.7888) ccw
  arc A269 (-44.6828, 75.2888) -> (-45.1828, 74.7888) centre (-44.6828, 74.7888) ccw
  arc A270 (-31.6828, 61.2888) -> (-31.1828, 61.7888) centre (-31.6828, 61.7888) ccw
  arc A271 (-31.1828, 74.7888) -> (-31.6828, 75.2888) centre (-31.6828, 74.7888) ccw
  line L272 (-45.1828, 80.8388) -> (-45.1828, 93.8388)
  line L273 (-31.1828, 80.8388) -> (-31.1828, 93.8388)
  line L274 (-44.6828, 80.3388) -> (-31.6828, 80.3388)
  line L275 (-44.6828, 94.3388) -> (-31.6828, 94.3388)
  arc A272 (-45.1828, 80.8388) -> (-44.6828, 80.3388) centre (-44.6828, 80.8388) ccw
  arc A273 (-44.6828, 94.3388) -> (-45.1828, 93.8388) centre (-44.6828, 93.8388) ccw
  arc A274 (-31.6828, 80.3388) -> (-31.1828, 80.8388) centre (-31.6828, 80.8388) ccw
  arc A275 (-31.1828, 93.8388) -> (-31.6828, 94.3388) centre (-31.6828, 93.8388) ccw
  line L276 (-45.1828, 99.8888) -> (-45.1828, 112.8888)
  line L277 (-31.1828, 99.8888) -> (-31.1828, 112.8888)
  line L278 (-44.6828, 99.3888) -> (-31.6828, 99.3888)
  line L279 (-44.6828, 113.3888) -> (-31.6828, 113.3888)
  arc A276 (-45.1828, 99.8888) -> (-44.6828, 99.3888) centre (-44.6828, 99.8888) ccw
  arc A277 (-44.6828, 113.3888) -> (-45.1828, 112.8888) centre (-44.6828, 112.8888) ccw
  arc A278 (-31.6828, 99.3888) -> (-31.1828, 99.8888) centre (-31.6828, 99.8888) ccw
  arc A279 (-31.1828, 112.8888) -> (-31.6828, 113.3888) centre (-31.6828, 112.8888) ccw
  line L280 (-45.1828, 118.9388) -> (-45.1828, 131.9388)
  line L281 (-31.1828, 118.9388) -> (-31.1828, 131.9388)
  line L282 (-44.6828, 118.4388) -> (-31.6828, 118.4388)
  line L283 (-44.6828, 132.4388) -> (-31.6828, 132.4388)
  arc A280 (-45.1828, 118.9388) -> (-44.6828, 118.4388) centre (-44.6828, 118.9388) ccw
  arc A281 (-44.6828, 132.4388) -> (-45.1828, 131.9388) centre (-44.6828, 131.9388) ccw
  arc A282 (-31.6828, 118.4388) -> (-31.1828, 118.9388) centre (-31.6828, 118.9388) ccw
  arc A283 (-31.1828, 131.9388) -> (-31.6828, 132.4388) centre (-31.6828, 131.9388) ccw
  line L284 (-45.1828, 137.9888) -> (-45.1828, 150.9888)
  line L285 (-31.1828, 137.9888) -> (-31.1828, 150.9888)
  line L286 (-44.6828, 137.4888) -> (-31.6828, 137.4888)
  line L287 (-44.6828, 151.4888) -> (-31.6828, 151.4888)
  arc A284 (-45.1828, 137.9888) -> (-44.6828, 137.4888) centre (-44.6828, 137.9888) ccw
  arc A285 (-44.6828, 151.4888) -> (-45.1828, 150.9888) centre (-44.6828, 150.9888) ccw
  arc A286 (-31.6828, 137.4888) -> (-31.1828, 137.9888) centre (-31.6828, 137.9888) ccw
  arc A287 (-31.1828, 150.9888) -> (-31.6828, 151.4888) centre (-31.6828, 150.9888) ccw
  line L288 (-45.1828, 157.0388) -> (-45.1828, 170.0388)
  line L289 (-31.1828, 157.0388) -> (-31.1828, 170.0388)
  line L290 (-44.6828, 156.5388) -> (-31.6828, 156.5388)
  line L291 (-44.6828, 170.5388) -> (-31.6828, 170.5388)
  arc A288 (-45.1828, 157.0388) -> (-44.6828, 156.5388) centre (-44.6828, 157.0388) ccw
  arc A289 (-44.6828, 170.5388) -> (-45.1828, 170.0388) centre (-44.6828, 170.0388) ccw
  arc A290 (-31.6828, 156.5388) -> (-31.1828, 157.0388) centre (-31.6828, 157.0388) ccw
  arc A291 (-31.1828, 170.0388) -> (-31.6828, 170.5388) centre (-31.6828, 170.0388) ccw
  line L292 (-45.1828, 176.0888) -> (-45.1828, 189.0888)
  line L293 (-31.1828, 176.0888) -> (-31.1828, 189.0888)
  line L294 (-44.6828, 175.5888) -> (-31.6828, 175.5888)
  line L295 (-44.6828, 189.5888) -> (-31.6828, 189.5888)
  arc A292 (-45.1828, 176.0888) -> (-44.6828, 175.5888) centre (-44.6828, 176.0888) ccw
  arc A293 (-44.6828, 189.5888) -> (-45.1828, 189.0888) centre (-44.6828, 189.0888) ccw
  arc A294 (-31.6828, 175.5888) -> (-31.1828, 176.0888) centre (-31.6828, 176.0888) ccw
  arc A295 (-31.1828, 189.0888) -> (-31.6828, 189.5888) centre (-31.6828, 189.0888) ccw
  line L296 (-45.1828, 195.1388) -> (-45.1828, 208.1388)
  line L297 (-31.1828, 195.1388) -> (-31.1828, 208.1388)
  line L298 (-44.6828, 194.6388) -> (-31.6828, 194.6388)
  line L299 (-44.6828, 208.6388) -> (-31.6828, 208.6388)
  arc A296 (-45.1828, 195.1388) -> (-44.6828, 194.6388) centre (-44.6828, 195.1388) ccw
  arc A297 (-44.6828, 208.6388) -> (-45.1828, 208.1388) centre (-44.6828, 208.1388) ccw
  arc A298 (-31.6828, 194.6388) -> (-31.1828, 195.1388) centre (-31.6828, 195.1388) ccw
  arc A299 (-31.1828, 208.1388) -> (-31.6828, 208.6388) centre (-31.6828, 208.1388) ccw
  line L300 (-45.1828, 214.1888) -> (-45.1828, 227.1888)
  line L301 (-31.1828, 214.1888) -> (-31.1828, 227.1888)
  line L302 (-44.6828, 213.6888) -> (-31.6828, 213.6888)
  line L303 (-44.6828, 227.6888) -> (-31.6828, 227.6888)
  arc A300 (-45.1828, 214.1888) -> (-44.6828, 213.6888) centre (-44.6828, 214.1888) ccw
  arc A301 (-44.6828, 227.6888) -> (-45.1828, 227.1888) centre (-44.6828, 227.1888) ccw
  arc A302 (-31.6828, 213.6888) -> (-31.1828, 214.1888) centre (-31.6828, 214.1888) ccw
  arc A303 (-31.1828, 227.1888) -> (-31.6828, 227.6888) centre (-31.6828, 227.1888) ccw
  line L304 (-45.1828, 233.2388) -> (-45.1828, 246.2388)
  line L305 (-31.1828, 233.2388) -> (-31.1828, 246.2388)
  line L306 (-44.6828, 232.7388) -> (-31.6828, 232.7388)
  line L307 (-44.6828, 246.7388) -> (-31.6828, 246.7388)
  arc A304 (-45.1828, 233.2388) -> (-44.6828, 232.7388) centre (-44.6828, 233.2388) ccw
  arc A305 (-44.6828, 246.7388) -> (-45.1828, 246.2388) centre (-44.6828, 246.2388) ccw
  arc A306 (-31.6828, 232.7388) -> (-31.1828, 233.2388) centre (-31.6828, 233.2388) ccw
  arc A307 (-31.1828, 246.2388) -> (-31.6828, 246.7388) centre (-31.6828, 246.2388) ccw
  line L308 (-45.1828, 268.9576) -> (-45.1828, 281.9576)
  line L309 (-31.1828, 268.9576) -> (-31.1828, 281.9576)
  line L310 (-44.6828, 268.4576) -> (-31.6828, 268.4576)
  line L311 (-44.6828, 282.4576) -> (-31.6828, 282.4576)
  arc A308 (-45.1828, 268.9576) -> (-44.6828, 268.4576) centre (-44.6828, 268.9576) ccw
  arc A309 (-44.6828, 282.4576) -> (-45.1828, 281.9576) centre (-44.6828, 281.9576) ccw
  arc A310 (-31.6828, 268.4576) -> (-31.1828, 268.9576) centre (-31.6828, 268.9576) ccw
  arc A311 (-31.1828, 281.9576) -> (-31.6828, 282.4576) centre (-31.6828, 281.9576) ccw
  line L312 (-44.1828, 260.5196) -> (-44.1828, 266.5196)
  line L313 (-29.1828, 260.5196) -> (-29.1828, 266.5196)
  line L314 (-43.6828, 260.0196) -> (-29.6828, 260.0196)
  line L315 (-43.6828, 267.0196) -> (-29.6828, 267.0196)
  arc A312 (-44.1828, 260.5196) -> (-43.6828, 260.0196) centre (-43.6828, 260.5196) ccw
  arc A313 (-43.6828, 267.0196) -> (-44.1828, 266.5196) centre (-43.6828, 266.5196) ccw
  arc A314 (-29.6828, 260.0196) -> (-29.1828, 260.5196) centre (-29.6828, 260.5196) ccw
  arc A315 (-29.1828, 266.5196) -> (-29.6828, 267.0196) centre (-29.6828, 266.5196) ccw
  line L316 (-44.1828, 284.3956) -> (-44.1828, 290.3956)
  line L317 (-29.1828, 284.3956) -> (-29.1828, 290.3956)
  line L318 (-43.6828, 283.8956) -> (-29.6828, 283.8956)
  line L319 (-43.6828, 290.8956) -> (-29.6828, 290.8956)
  arc A316 (-44.1828, 284.3956) -> (-43.6828, 283.8956) centre (-43.6828, 284.3956) ccw
  arc A317 (-43.6828, 290.8956) -> (-44.1828, 290.3956) centre (-43.6828, 290.3956) ccw
  arc A318 (-29.6828, 283.8956) -> (-29.1828, 284.3956) centre (-29.6828, 284.3956) ccw
  arc A319 (-29.1828, 290.3956) -> (-29.6828, 290.8956) centre (-29.6828, 290.3956) ccw
  line L320 (-45.1828, 328.4888) -> (-45.1828, 341.4888)
  line L321 (-31.1828, 328.4888) -> (-31.1828, 341.4888)
  line L322 (-44.6828, 327.9888) -> (-31.6828, 327.9888)
  line L323 (-44.6828, 341.9888) -> (-31.6828, 341.9888)
  arc A320 (-45.1828, 328.4888) -> (-44.6828, 327.9888) centre (-44.6828, 328.4888) ccw
  arc A321 (-44.6828, 341.9888) -> (-45.1828, 341.4888) centre (-44.6828, 341.4888) ccw
  arc A322 (-31.6828, 327.9888) -> (-31.1828, 328.4888) centre (-31.6828, 328.4888) ccw
  arc A323 (-31.1828, 341.4888) -> (-31.6828, 341.9888) centre (-31.6828, 341.4888) ccw
  line L324 (-26.1328, 21.3076) -> (-26.1328, 34.3076)
  line L325 (-12.1328, 21.3076) -> (-12.1328, 34.3076)
  line L326 (-25.6328, 20.8076) -> (-12.6328, 20.8076)
  line L327 (-25.6328, 34.8076) -> (-12.6328, 34.8076)
  arc A324 (-26.1328, 21.3076) -> (-25.6328, 20.8076) centre (-25.6328, 21.3076) ccw
  arc A325 (-25.6328, 34.8076) -> (-26.1328, 34.3076) centre (-25.6328, 34.3076) ccw
  arc A326 (-12.6328, 20.8076) -> (-12.1328, 21.3076) centre (-12.6328, 21.3076) ccw
  arc A327 (-12.1328, 34.3076) -> (-12.6328, 34.8076) centre (-12.6328, 34.3076) ccw
  line L328 (-26.1328, 45.1201) -> (-26.1328, 58.1201)
  line L329 (-12.1328, 45.1201) -> (-12.1328, 58.1201)
  line L330 (-25.6328, 44.6201) -> (-12.6328, 44.6201)
  line L331 (-25.6328, 58.6201) -> (-12.6328, 58.6201)
  arc A328 (-26.1328, 45.1201) -> (-25.6328, 44.6201) centre (-25.6328, 45.1201) ccw
  arc A329 (-25.6328, 58.6201) -> (-26.1328, 58.1201) centre (-25.6328, 58.1201) ccw
  arc A330 (-12.6328, 44.6201) -> (-12.1328, 45.1201) centre (-12.6328, 45.1201) ccw
  arc A331 (-12.1328, 58.1201) -> (-12.6328, 58.6201) centre (-12.6328, 58.1201) ccw
  line L332 (-26.1328, 68.9326) -> (-26.1328, 81.9326)
  line L333 (-12.1328, 68.9326) -> (-12.1328, 81.9326)
  line L334 (-25.6328, 68.4326) -> (-12.6328, 68.4326)
  line L335 (-25.6328, 82.4326) -> (-12.6328, 82.4326)
  arc A332 (-26.1328, 68.9326) -> (-25.6328, 68.4326) centre (-25.6328, 68.9326) ccw
  arc A333 (-25.6328, 82.4326) -> (-26.1328, 81.9326) centre (-25.6328, 81.9326) ccw
  arc A334 (-12.6328, 68.4326) -> (-12.1328, 68.9326) centre (-12.6328, 68.9326) ccw
  arc A335 (-12.1328, 81.9326) -> (-12.6328, 82.4326) centre (-12.6328, 81.9326) ccw
  line L336 (-26.1328, 140.3701) -> (-26.1328, 153.3701)
  line L337 (-12.1328, 140.3701) -> (-12.1328, 153.3701)
  line L338 (-25.6328, 139.8701) -> (-12.6328, 139.8701)
  line L339 (-25.6328, 153.8701) -> (-12.6328, 153.8701)
  arc A336 (-26.1328, 140.3701) -> (-25.6328, 139.8701) centre (-25.6328, 140.3701) ccw
  arc A337 (-25.6328, 153.8701) -> (-26.1328, 153.3701) centre (-25.6328, 153.3701) ccw
  arc A338 (-12.6328, 139.8701) -> (-12.1328, 140.3701) centre (-12.6328, 140.3701) ccw
  arc A339 (-12.1328, 153.3701) -> (-12.6328, 153.8701) centre (-12.6328, 153.3701) ccw
  line L340 (-25.1328, 93.8701) -> (-25.1328, 99.8701)
  line L341 (-10.1328, 93.8701) -> (-10.1328, 99.8701)
  line L342 (-24.6328, 93.3701) -> (-10.6328, 93.3701)
  line L343 (-24.6328, 100.3701) -> (-10.6328, 100.3701)